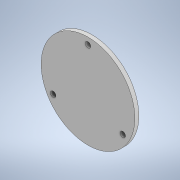
# Autodesk Inventor part: Griff_Deckel
Saved by Autodesk Inventor 2022 (Build 260153000, 153)
## iProperties
Created: 2021-06-17
Part Number: Griff_Deckel
Material: Generic
Document SubType Name: Modeling
Designer: Cornee
Density: 1 g/cm^3
Appearance: Default
Author: Cornee
Autodesk Inventor part; units mm, degrees
ref_plane "YZ Plane" through (0, 0, 0) normal (1, 0, 0) x (0, 1, 0)
ref_plane "XZ Plane" through (0, 0, 0) normal (0, 1, 0) x (-1, 0, 0)
ref_plane "XY Plane" through (0, 0, 0) normal (0, 0, 1) x (1, 0, 0)
sketch "Sketch1" plane through (0, 0, 0) normal (0, 0, 1) x (1, 0, 0)
  circle A0 centre (0, 0) radius 35
  circle A1 centre (0, 30) radius 2.05
  circle A2 centre (-25.981, -15) radius 2.05
  circle A3 centre (25.981, -15) radius 2.05
  dimension "d0" = 70
  dimension "d1" = 4.1
  dimension "d2" = 30
  dimension "d3" = 4.1
  dimension "d4" = 4.1
  dimension "d5" = 15
  dimension "d6" = 25.981
  dimension "d7" = 25.981
  constraints: 4 centre point, 1 coincident, 1 horizontal alignment, 1 vertical alignment
  measures "d0" diameter of A0
  measures "d1" diameter of A1
  measures "d2" distance of point (0, 0) A1.centre
  measures "d3" diameter of A2
  measures "d4" diameter of A3
  measures "d5" vertical distance of A2.centre point (0, 0)
  measures "d6" horizontal distance of point (0, 0) A2.centre
  measures "d7" horizontal distance of point (0, 0) A3.centre
extrude "Extrusion1" add sketch "Sketch1" along normal blind 3
equation "\"d7\" = d6"
body "Solid1"
